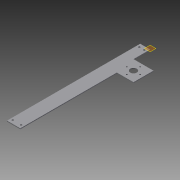
# Autodesk Inventor part: Cim Mount
Saved by Autodesk Inventor 2013 (Build 170138000, 138)
## iProperties
Created: 2013-01-24
Part Number: Cim Mount
Material: Generic
Document SubType Name: Modeling
Designer: actoennies
Density: 1 g/cm^3
Author: actoennies
Autodesk Inventor part; units mm, degrees
ref_plane "YZ Plane" through (0, 0, 0) normal (1, 0, 0) x (0, 1, 0)
ref_plane "XZ Plane" through (0, 0, 0) normal (0, 1, 0) x (-1, 0, 0)
ref_plane "XY Plane" through (0, 0, 0) normal (0, 0, 1) x (1, 0, 0)
sketch "Sketch1" plane through (0, 0, 0) normal (0, 1, 0) x (-1, 0, 0)
  line L0 (0, 0) -> (0, 63.5)
  line L1 (0, 63.5) -> (-63.5, 63.5)
  line L2 (-63.5, 63.5) -> (-63.5, 139.7)
  line L3 (-63.5, 139.7) -> (0, 139.7)
  line L4 (0, 139.7) -> (0, 495.3)
  line L5 (0, 495.3) -> (50.8, 495.3)
  line L6 (50.8, 495.3) -> (50.8, 0)
  line L7 (50.8, 0) -> (0, 0)
  circle A0 centre (-25.4, 101.6) radius 25.4 construction
  circle A1 centre (-25.4, 127) radius 2.5527
  circle A2 centre (-50.8, 101.6) radius 2.5527
  circle A3 centre (-25.4, 76.2) radius 2.5527
  circle A4 centre (0, 101.6) radius 2.5527
  dimension "d6" = 50.8
  dimension "d1" = 63.5
  dimension "d2" = 63.5
  dimension "d3" = 76.2
  dimension "d4" = 355.6
  dimension "d5" = 50.8
  dimension "d30" = 101.6
  dimension "d31" = 38.1
  dimension "d32" = 5.1054
  dimension "d35" = 360
  constraints: 16 end point, 4 centre point, 4 perpendicular, 3 parallel, 1 vertical, 1 vertical alignment, 11 other
  measures "d1" distance of L0.start L0.end
  measures "d2" distance of L0.end L1.end
  measures "d3" distance of L1.end L2.end
  measures "d4" distance of L3.end L4.end
  measures "d5" distance of L4.end L5.end
  measures "d30" distance from line of L7 point (-25.4, 101.6)
  measures "d31" distance from line of L2 point (-25.4, 101.6)
  measures "d32" diameter of A1
ref_plane "Work Plane2" through (0, 6.35, 0) normal (0, 1, 0) x (1, 0, 0)
ref_plane "Work Plane1" through (0, 6.35, 0) normal (0, 1, 0) x (1, 0, 0)
extrude "Extrusion4" add sketch "Sketch1" along normal blind 3.175
sketch "Sketch4" plane through (0, 3.175, 0) normal (0, 1, 0) x (1, 0, 0)
  line L0 (0, -63.5) -> (0, 0) projected
  line L1 (0, 0) -> (-50.8, 0) projected
  line L2 (-50.8, 0) -> (-50.8, -495.3) projected
  line L3 (-50.8, -495.3) -> (0, -495.3) projected
  line L4 (0, -495.3) -> (0, -139.7) projected
  circle A0 centre (25.4, -101.6) radius 12.7
  circle A1 centre (-41.275, -12.7) radius 3.3782
  circle A2 centre (-9.525, -12.7) radius 3.3782
  circle A3 centre (-41.275, -482.6) radius 3.3782
  circle A4 centre (-9.525, -482.6) radius 3.3782
  line L5 (63.5, -139.7) -> (63.5, -63.5) projected
  dimension "d39" = 25.4
  dimension "d40" = 6.7564
  dimension "d41" = 6.7564
  dimension "d42" = 6.7564
  dimension "d43" = 6.7564
  dimension "d44" = 12.7
  dimension "d45" = 12.7
  dimension "d46" = 9.525
  dimension "d47" = 9.525
  dimension "d48" = 12.7
  dimension "d49" = 9.525
  dimension "d50" = 12.7
  dimension "d51" = 9.525
  dimension "d54" = 38.1
  constraints: 5 centre point
  measures "d39" diameter of A0
  measures "d40" diameter of A1
  measures "d41" diameter of A2
  measures "d42" diameter of A3
  measures "d43" diameter of A4
  measures "d44" distance from line of L3 A3.centre
  measures "d45" distance from line of L3 A4.centre
  measures "d46" distance from line of L2 A3.centre
  measures "d47" distance from line of L4 A4.centre
  measures "d48" distance from line of L1 A1.centre
  measures "d49" distance from line of A1.centre L2
  measures "d50" distance from line of A2.centre L1
  measures "d51" distance from line of L0 A2.centre
  measures "d54" distance from line of A0.centre L5
extrude "Extrusion5" cut sketch "Sketch4" against normal blind 3.175
body "Solid1"
